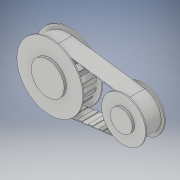
# Autodesk Inventor part: chain sproket
Saved by Autodesk Inventor 2018 (Build 220112000, 112)
## iProperties
Created: 2021-03-17
Part Number: chain sproket
Material: Generic
Document SubType Name: Modeling
Designer: Jyoti Soni
Density: 1 g/cm^3
Appearance: Default
Author: Jyoti Soni
Autodesk Inventor part; units mm, degrees
ref_plane "YZ Plane" through (0, 0, 0) normal (1, 0, 0) x (0, 1, 0)
sketch "Sketch1" plane through (0, 0, 0) normal (0, 0, 1) x (1, 0, 0)
  circle A0 centre (0, 0) radius 75
  circle A1 centre (167.5, 0) radius 50
  dimension "d0" = 150
  dimension "d1" = 100
  dimension "d2" = 167.5
  constraints: 2 centre point, 1 coincident
  measures "d0" diameter of A0
  measures "d1" diameter of A1
  measures "d2" distance of A1.centre point (0, 0)
extrude "Extrusion1" add sketch "Sketch1" along normal blind 2.5
ref_plane "Work Plane1" through (0, 0, 1.25) normal (0, 0, 1) x (1, 0, 0)
sketch "Sketch2" plane through (0, 0, 1.25) normal (0, 0, 1) x (1, 0, 0)
  point P0 (0, 0)
ref_plane "Work Plane2" through (0, 0, 42.5) normal (0, 0, 1) x (1, 0, 0)
sketch "Sketch3" plane through (0, 0, 42.5) normal (0, 0, 1) x (1, 0, 0)
  circle A0 centre (0, 0) radius 75 projected
  circle A1 centre (167.5, 0) radius 50 projected
extrude "Extrusion2" add sketch "Sketch3" along normal blind 2.5
sketch "Sketch5" plane through (0, 0, 2.5) normal (0, 0, 1) x (1, 0, 0)
  arc A0 (8.591182, 61.906717) -> (0, 62.5) centre (0, 0) ccw
  arc A1 (8.773822, 63.395742) -> (0, 64) centre (0, 0) ccw
  line L0 (0, 64) -> (0, 62.5)
  line L1 (8.773822, 63.395742) -> (8.591182, 61.906717)
  dimension "d12" = 125
  dimension "d20" = 1.5
  constraints: 4 end point, 4 point on circle, 2 centre point, 1 coincident, 1 vertical
  measures "d12" diameter of A0
  measures "d20" radial gap between concentric circles of A0 A1
extrude "Extrusion4" add sketch "Sketch5" along normal blind 40
sketch "Sketch6" plane through (167.5, 0, 2.5) normal (0, 0, 1) x (1, 0, 0)
  arc A0 (0, 40) -> (-8.314899, 39.126237) centre (0, 0) ccw
  arc A1 (0, 41.5) -> (-8.716924, 40.574194) centre (0, 0) ccw
  line L0 (0, 40) -> (0, 41.5)
  line L1 (-8.314899, 39.126237) -> (-8.716924, 40.574194)
  point P0 (-167.5, 0)
  dimension "d15" = 80
  dimension "d25" = 1.5
  constraints: 4 end point, 4 point on circle, 2 centre point, 1 vertical
  measures "d15" diameter of A0
  measures "d25" radial gap between concentric circles of A1 A0
extrude "Extrusion5" add sketch "Sketch6" along normal blind 40
pattern_circular "Circular Pattern1" count 18 over 360 about axis through (0, 0, 42.5) along (0, 0, 1) of "Extrusion4"
pattern_circular "Circular Pattern2" count 12 over 360 about axis through (167.5, 0, 0) along (0, 0, 1) of "Extrusion5"
sketch "Sketch8" plane through (0, 0, 2.5) normal (0, 0, 1) x (1, 0, 0)
  arc A0 (8.773822, 63.395742) -> (0, 64) centre (0, 0) ccw construction
  arc A1 (-13.437925, 62.573334) -> (-21.889289, 60.140328) centre (0, 0) ccw construction
  arc A2 (167.5, 41.5) -> (158.783076, 40.574194) centre (167.5, 0) ccw construction
  arc A3 (188.25, 35.940054) -> (180.238019, 39.496745) centre (167.5, 0) ccw construction
  arc A4 (173.074627, -41.12388) -> (173.074627, 41.12388) centre (167.5, 0) ccw
  line L0 (0, 64) -> (0, 62.5)
  arc A5 (8.597015, 63.41996) -> (8.597015, -63.41996) centre (0, 0) ccw
  line L1 (173.074627, 41.12388) -> (8.597015, 63.41996)
  line L2 (8.597015, -63.41996) -> (173.074627, -41.12388)
  line L3 (8.798507, 64.906365) -> (173.276119, 42.610286)
  arc A6 (173.276119, -42.610286) -> (173.276119, 42.610286) centre (167.5, 0) ccw
  line L4 (173.276119, -42.610286) -> (8.798507, -64.906365)
  arc A7 (8.798507, 64.906365) -> (8.798507, -64.906365) centre (0, 0) ccw
  dimension "d29" = 1.5
  constraints: 9 point on circle, 8 end point, 4 centre point, 4 tangent, 2 coincident, 1 concentric, 3 other
  measures "d29" distance between parallel lines of L3 L1
extrude "Extrusion8" add sketch "Sketch8" along normal blind 40
sketch "Sketch9" plane through (0, 0, 45) normal (0, 0, 1) x (1, 0, 0)
  circle A0 centre (0, 0) radius 37.5
  circle A1 centre (167.5, 0) radius 25
  circle A2 centre (167.5, 0) radius 50 construction
  dimension "d34" = 75
  dimension "d35" = 50
  constraints: 2 centre point, 1 coincident, 1 concentric
  measures "d34" diameter of A0
  measures "d35" diameter of A1
extrude "Extrusion9" add sketch "Sketch9" along normal blind 5
sketch "Sketch10" plane through (0, 0, 42.5) normal (0, 0, 1) x (1, 0, 0)
  line L0 (47.345054, 58.167395) -> (145.439211, 44.870052) construction
  line L1 (145.439211, -44.870052) -> (47.345054, -58.167395) construction
  line L2 (47.345054, -58.167395) -> (8.597015, -63.41996) construction
  line L3 (8.597015, 63.41996) -> (47.345054, 58.167395) construction
  line L4 (145.439211, 44.870052) -> (173.074627, 41.12388) construction
  line L5 (173.074627, -41.12388) -> (145.439211, -44.870052) construction
  line L6 (8.591182, 61.906717) -> (8.773822, 63.395742) construction
  line L7 (10.814086, 61.605702) -> (11.015579, 63.092107)
  line L8 (13.752337, 61.207401) -> (13.95383, 62.693807)
  line L9 (47.345054, 58.167395) -> (8.597015, 63.41996) construction
  line L10 (17.94755, 60.638711) -> (18.149043, 62.125117)
  line L11 (22.637251, 60.00299) -> (22.838743, 61.489395)
  line L12 (29.859387, 59.023979) -> (30.06088, 60.510384)
  line L13 (34.20316, 58.435151) -> (34.404653, 59.921556)
  line L14 (38.686404, 57.827416) -> (38.887897, 59.313821)
  line L15 (42.91005, 57.254871) -> (43.111543, 58.741277)
  line L16 (145.439211, 44.870052) -> (47.345054, 58.167395) construction
  line L17 (47.345054, 58.167395) -> (47.143562, 56.68099)
  line L18 (52.621536, 55.938412) -> (52.823028, 57.424818)
  line L19 (58.070367, 55.199785) -> (58.271859, 56.686191)
  line L20 (66.111922, 54.109697) -> (66.313414, 55.596102)
  line L21 (73.102561, 53.162067) -> (73.304054, 54.648473)
  line L22 (81.258461, 52.056479) -> (81.459954, 53.542884)
  line L23 (93.440737, 50.405087) -> (93.642229, 51.891492)
  line L24 (106.128736, 48.685141) -> (106.330229, 50.171546)
  line L25 (115.483387, 47.417053) -> (115.684879, 48.903458)
  line L26 (124.316819, 46.21962) -> (124.518312, 47.706025)
  line L27 (134.920455, 44.782224) -> (135.121947, 46.268629)
  line L28 (145.630628, 44.844105) -> (145.429135, 43.357699)
  line L29 (156.768513, 41.820568) -> (156.970006, 43.306973)
  line L30 (173.074627, 41.12388) -> (172.873134, 39.637475)
  line L31 (13.752337, 61.207401) -> (10.814086, 61.605702)
  line L32 (22.637251, 60.00299) -> (17.94755, 60.638711)
  line L33 (42.91005, 57.254871) -> (38.686404, 57.827416)
  line L34 (34.20316, 58.435151) -> (29.859387, 59.023979)
  line L35 (52.621536, 55.938412) -> (47.143562, 56.68099)
  line L36 (66.111922, 54.109697) -> (58.070367, 55.199785)
  line L37 (81.258461, 52.056479) -> (73.102561, 53.162067)
  line L38 (106.128736, 48.685141) -> (93.440737, 50.405087)
  line L39 (145.237719, 43.383647) -> (134.920455, 44.782224)
  line L40 (124.316819, 46.21962) -> (115.483387, 47.417053)
  line L41 (172.873134, 39.637475) -> (156.768513, 41.820568)
  line L42 (145.429135, 43.357699) -> (145.237719, 43.383647)
  line L43 (8.597015, -63.188513) -> (8.597015, -63.41996)
  line L44 (14.854971, -61.057932) -> (15.056464, -62.544337)
  line L45 (24.696959, -61.237501) -> (24.495467, -59.751096)
  line L46 (36.962925, -59.574765) -> (36.761432, -58.088359)
  line L47 (50.958382, -57.677583) -> (50.756889, -56.191178)
  line L48 (68.90142, -53.731561) -> (69.102912, -55.217967)
  line L49 (86.865601, -51.296392) -> (87.067093, -52.782797)
  line L50 (109.559724, -48.220046) -> (109.761217, -49.706452)
  line L51 (119.469093, -46.876763) -> (119.670585, -48.363168)
  line L52 (138.869835, -44.246858) -> (139.071328, -45.733263)
  line L53 (148.898428, -42.887413) -> (149.607739, -44.30498)
  line L54 (157.548081, -41.714892) -> (157.906487, -43.180027)
  line L55 (173.203664, -39.592669) -> (173.074627, -41.12388)
  line L56 (15.056464, -62.544337) -> (24.696959, -61.237501) construction
  line L57 (8.597015, -63.41996) -> (15.056464, -62.544337) construction
  line L58 (14.854971, -61.057932) -> (24.495467, -59.751096)
  line L59 (36.761432, -58.088359) -> (47.143562, -56.68099)
  line L60 (24.696959, -61.237501) -> (26.883507, -60.972532) construction
  line L61 (31.266816, -60.441357) -> (36.962925, -59.751096) construction
  line L62 (47.143562, -56.68099) -> (50.756889, -56.191178)
  line L63 (68.90142, -53.731561) -> (86.865601, -51.296392)
  line L64 (109.559724, -48.220046) -> (119.469093, -46.876763)
  line L65 (138.869835, -44.246858) -> (145.237719, -43.383647)
  line L66 (145.237719, -43.383647) -> (148.898428, -42.887413)
  line L67 (157.548081, -41.714892) -> (172.873134, -39.637475)
  line L68 (173.074627, -41.12388) -> (157.895602, -43.13553) construction
  line L69 (149.607739, -44.30498) -> (139.071328, -45.733263) construction
  line L70 (109.761217, -49.706452) -> (119.670585, -48.363168)
  line L71 (15.056464, -62.544337) -> (24.696959, -61.237501)
  line L72 (11.015579, 63.092107) -> (13.95383, 62.693807)
  line L73 (18.149043, 62.125117) -> (22.838743, 61.489395)
  line L74 (30.06088, 60.510384) -> (34.404653, 59.921556)
  line L75 (47.345054, 58.167395) -> (52.823028, 57.424818)
  line L76 (58.271859, 56.686191) -> (66.313414, 55.596102)
  line L77 (73.304054, 54.648473) -> (81.459954, 53.542884)
  line L78 (93.642229, 51.891492) -> (106.330229, 50.171546)
  line L79 (115.684879, 48.903458) -> (124.518312, 47.706025)
  line L80 (135.121947, 46.268629) -> (145.630628, 44.844105)
  line L81 (173.074627, 41.12388) -> (145.439211, 44.870052)
  line L82 (156.970006, 43.306973) -> (173.074627, 41.12388)
  point P0 (0, 0)
  dimension "d45" = 10
  constraints: 146 end point, 27 perpendicular, 18 point on line, 10 parallel, 6 collinear, 1 vertical, 21 other
  measures "d45" distance of L50.start L51.start
extrude "Extrusion10" add sketch "Sketch10" against normal blind 38.3375 separate body contours L64 L51 L70 L50
pattern_linear "Rectangular Pattern1" count 5 spacing 25 along (-0.9909369, -0.1343284, 0) of "Extrusion10" bodies 2
pattern_linear "Rectangular Pattern2" count 2 spacing 25 along (0.9909369, 0.1343284, 0) of "Extrusion10" bodies 2
sketch "Sketch11" plane through (0, 0, 42.5) normal (0, 0, 1) x (1, 0, 0)
  point P0 (0, 0)
sketch "Sketch12" plane through (0, 0, 42.5) normal (0, 0, 1) x (1, 0, 0)
  line L0 (47.345054, 58.167395) -> (145.439211, 44.870052) construction
  line L1 (145.439211, 44.870052) -> (145.439211, 43.356333)
  line L2 (145.439211, 43.356333) -> (135.529843, 44.699617)
  line L3 (135.529843, 44.699617) -> (135.731335, 46.186022)
  line L4 (173.074627, 41.12388) -> (145.439211, 44.870052) construction
  line L5 (135.731335, 46.186022) -> (145.439211, 44.870052)
  point P0 (0, 0)
  dimension "d54" = 10
  dimension "d55" = 1.5
  constraints: 8 end point, 1 collinear, 1 parallel, 1 perpendicular, 1 point on line, 1 vertical
  measures "d54" distance of L1.end L2.end
  measures "d55" distance of L2.end L3.end
extrude "Extrusion11" add sketch "Sketch12" against normal blind 40 bodies 1
pattern_linear "Rectangular Pattern3" count 5 spacing 25 along (-0.9909369, 0.1343284, 0) of "Extrusion11" bodies 1
body "Solid1"
body "Solid3"
